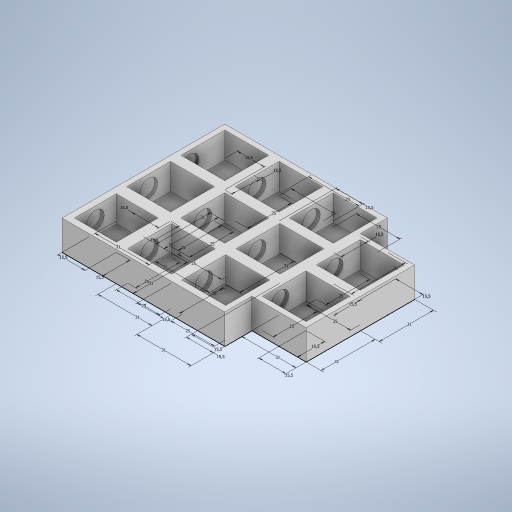
# Autodesk Inventor part: новая коробка
Saved by Autodesk Inventor 2024.2 (Build 282272000, 272)
## iProperties
Created: 2026-01-06
Part Number: новая коробка
Material: Типовые
Document SubType Name: Modeling
Designer: User
Density: 1 g/cm^3
Appearance: По умолчанию
Author: User
Autodesk Inventor part; units mm, degrees
ref_plane "YZ Plane" through (0, 0, 0) normal (1, 0, 0) x (0, 1, 0)
ref_plane "XZ Plane" through (0, 0, 0) normal (0, 1, 0) x (-1, 0, 0)
ref_plane "XY Plane" through (0, 0, 0) normal (0, 0, 1) x (1, 0, 0)
sketch "Эскиз1" plane through (0, 0, 0) normal (0, 1, 0) x (-1, 0, 0)
  line L0 (-12.5, -12.5) -> (12.5, -12.5)
  line L1 (12.5, -12.5) -> (12.5, 12.5)
  line L2 (12.5, 12.5) -> (-12.5, 12.5)
  line L3 (-12.5, 12.5) -> (-12.5, -12.5)
  line L4 (-12.5, -12.5) -> (12.5, 12.5) construction
  line L5 (12.5, -12.5) -> (-12.5, 12.5) construction
  line L6 (-15.5, -15.5) -> (15.5, -15.5)
  line L7 (15.5, -15.5) -> (15.5, 15.5)
  line L8 (15.5, 15.5) -> (-15.5, 15.5)
  line L9 (-15.5, 15.5) -> (-15.5, -15.5)
  line L10 (-15.5, -15.5) -> (15.5, 15.5) construction
  line L11 (15.5, -15.5) -> (-15.5, 15.5) construction
  line L12 (15.5, 15.5) -> (46.5, 15.5)
  line L13 (46.5, 15.5) -> (46.5, -15.5)
  line L14 (46.5, -15.5) -> (15.5, -15.5)
  line L15 (15.5, -15.5) -> (15.5, 15.5)
  line L16 (-15.5, 15.5) -> (-46.5, 15.5)
  line L17 (-46.5, 15.5) -> (-46.5, -15.5)
  line L18 (-46.5, -15.5) -> (-15.5, -15.5)
  line L19 (-15.5, -15.5) -> (-15.5, 15.5)
  line L20 (46.5, -15.5) -> (13.5, -15.5)
  line L21 (13.5, -15.5) -> (13.5, -46.5)
  line L22 (13.5, -46.5) -> (46.5, -46.5)
  line L23 (46.5, -46.5) -> (46.5, -15.5)
  line L24 (-15.5, -15.5) -> (13.5, -15.5)
  line L25 (13.5, -15.5) -> (13.5, -46.5)
  line L26 (13.5, -46.5) -> (-15.5, -46.5)
  line L27 (-15.5, -46.5) -> (-15.5, -15.5)
  line L28 (-15.5, -15.5) -> (-46.5, -15.5)
  line L29 (-46.5, -15.5) -> (-46.5, -46.5)
  line L30 (-46.5, -46.5) -> (-15.5, -46.5)
  line L31 (-15.5, -46.5) -> (-15.5, -15.5)
  line L32 (46.5, 15.5) -> (15.5, 15.5)
  line L33 (15.5, 15.5) -> (15.5, 46.5)
  line L34 (15.5, 46.5) -> (46.5, 46.5)
  line L35 (46.5, 46.5) -> (46.5, 15.5)
  line L36 (15.5, 46.5) -> (-15.5, 46.5)
  line L37 (-15.5, 46.5) -> (-15.5, 15.5)
  line L38 (-15.5, 15.5) -> (15.5, 15.5)
  line L39 (15.5, 15.5) -> (15.5, 46.5)
  line L40 (-15.5, 46.5) -> (-46.5, 46.5)
  line L41 (-46.5, 46.5) -> (-46.5, 15.5)
  line L42 (-46.5, 15.5) -> (-15.5, 15.5)
  line L43 (-15.5, 15.5) -> (-15.5, 46.5)
  line L44 (-46.5, 0) -> (-77.5, 0)
  line L45 (-77.5, 0) -> (-77.5, -31)
  line L46 (-77.5, -31) -> (-46.5, -31)
  line L47 (-46.5, -31) -> (-46.5, 0)
  line L48 (-46.5, 0) -> (-77.5, 0)
  line L49 (-77.5, 0) -> (-77.5, 31)
  line L50 (-77.5, 31) -> (-46.5, 31)
  line L51 (-46.5, 31) -> (-46.5, 0)
  line L52 (-12.5, 17.9528) -> (12.5, 17.9528)
  line L53 (12.5, 17.9528) -> (12.5, 42.9528)
  line L54 (12.5, 42.9528) -> (-12.5, 42.9528)
  line L55 (-12.5, 42.9528) -> (-12.5, 17.9528)
  line L56 (-12.5, 17.9528) -> (12.5, 42.9528) construction
  line L57 (12.5, 17.9528) -> (-12.5, 42.9528) construction
  line L58 (19.0472, 19.0472) -> (42.9528, 19.0472)
  line L59 (42.9528, 19.0472) -> (42.9528, 42.9528)
  line L60 (42.9528, 42.9528) -> (19.0472, 42.9528)
  line L61 (19.0472, 42.9528) -> (19.0472, 19.0472)
  line L62 (19.0472, 19.0472) -> (42.9528, 42.9528) construction
  line L63 (42.9528, 19.0472) -> (19.0472, 42.9528) construction
  line L64 (-43.5, 17.9528) -> (-18.5, 17.9528)
  line L65 (-18.5, 17.9528) -> (-18.5, 42.9528)
  line L66 (-18.5, 42.9528) -> (-43.5, 42.9528)
  line L67 (-43.5, 42.9528) -> (-43.5, 17.9528)
  line L68 (-43.5, 17.9528) -> (-18.5, 42.9528) construction
  line L69 (-18.5, 17.9528) -> (-43.5, 42.9528) construction
  line L70 (-43.5, -13.0472) -> (-18.5, -13.0472)
  line L71 (-18.5, -13.0472) -> (-18.5, 11.9528)
  line L72 (-18.5, 11.9528) -> (-43.5, 11.9528)
  line L73 (-43.5, 11.9528) -> (-43.5, -13.0472)
  line L74 (-43.5, -13.0472) -> (-18.5, 11.9528) construction
  line L75 (-18.5, -13.0472) -> (-43.5, 11.9528) construction
  line L76 (-43.5, -43.5) -> (-18.5, -43.5)
  line L77 (-18.5, -43.5) -> (-18.5, -18.5)
  line L78 (-18.5, -18.5) -> (-43.5, -18.5)
  line L79 (-43.5, -18.5) -> (-43.5, -43.5)
  line L80 (-43.5, -43.5) -> (-18.5, -18.5) construction
  line L81 (-18.5, -43.5) -> (-43.5, -18.5) construction
  line L82 (18.5, -43.5646) -> (43.5, -43.5646)
  line L83 (43.5, -43.5646) -> (43.5, -18.5)
  line L84 (43.5, -18.5) -> (18.5, -18.5)
  line L85 (18.5, -18.5) -> (18.5, -43.5646)
  line L86 (18.5, -43.5646) -> (43.5, -18.5) construction
  line L87 (43.5, -43.5646) -> (18.5, -18.5) construction
  line L88 (-12.5, -43.5) -> (12.5, -43.5)
  line L89 (12.5, -43.5) -> (12.5, -18.5)
  line L90 (12.5, -18.5) -> (-12.5, -18.5)
  line L91 (-12.5, -18.5) -> (-12.5, -43.5)
  line L92 (-12.5, -43.5) -> (12.5, -18.5) construction
  line L93 (12.5, -43.5) -> (-12.5, -18.5) construction
  line L94 (18.5, -12.5) -> (43.5, -12.5)
  line L95 (43.5, -12.5) -> (43.5, 12.5)
  line L96 (43.5, 12.5) -> (18.5, 12.5)
  line L97 (18.5, 12.5) -> (18.5, -12.5)
  line L98 (18.5, -12.5) -> (43.5, 12.5) construction
  line L99 (43.5, -12.5) -> (18.5, 12.5) construction
  line L100 (-74.5, -28) -> (-49.5, -28)
  line L101 (-49.5, -28) -> (-49.5, -3)
  line L102 (-49.5, -3) -> (-74.5, -3)
  line L103 (-74.5, -3) -> (-74.5, -28)
  line L104 (-74.5, -28) -> (-49.5, -3) construction
  line L105 (-49.5, -28) -> (-74.5, -3) construction
  line L106 (-74.5, 28) -> (-49.5, 28)
  line L107 (-49.5, 28) -> (-49.5, 3)
  line L108 (-49.5, 3) -> (-74.5, 3)
  line L109 (-74.5, 3) -> (-74.5, 28)
  line L110 (-74.5, 28) -> (-49.5, 3) construction
  line L111 (-49.5, 28) -> (-74.5, 3) construction
  point P0 (0, 0)
  point P1 (0, 30.4528)
  point P2 (31, 31)
  point P3 (-31, 30.4528)
  point P4 (-31, -0.5472)
  point P5 (-31, -31)
  point P6 (31, -31.0323)
  point P7 (0, -31)
  point P8 (31, 0)
  point P9 (-62, -15.5)
  point P10 (-62, 0)
  point P11 (-77.5, -15.5)
  point P12 (-62, 15.5)
  point P13 (-62, 31)
  point P14 (-46.5, -31)
  point P15 (46.5, 31)
  point P16 (30, -46.5)
  point P17 (-31, -46.5)
  point P18 (31, 15.5)
  dimension "d0" = 25
  dimension "d1" = 25
  dimension "d2" = 31
  dimension "d3" = 31
  dimension "d4" = 31
  dimension "d5" = 31
  dimension "d6" = 31
  dimension "d7" = 31
  dimension "d8" = 31
  dimension "d9" = 29
  dimension "d10" = 31
  dimension "d11" = 31
  dimension "d12" = 31
  dimension "d13" = 31
  dimension "d14" = 31
  dimension "d15" = 25
  dimension "d16" = 25
  dimension "d17" = 15.5
  dimension "d19" = 25
  dimension "d20" = 15.5
  dimension "d41" = 15.5
  dimension "d42" = 15.5
  dimension "d43" = 15.5
  dimension "d44" = 15.5
  dimension "d45" = 15.5
  dimension "d46" = 15.5
  dimension "d47" = 15.5
  dimension "d48" = 25
  dimension "d49" = 25
  dimension "d50" = 25
  dimension "d51" = 25
  dimension "d52" = 25
  dimension "d53" = 25
  dimension "d54" = 25
  dimension "d55" = 25
  dimension "d56" = 15.5
  dimension "d57" = 15.5
  dimension "d58" = 15.5
  dimension "d59" = 15.5
  dimension "d60" = 15.5
  dimension "d61" = 15.5
  constraints: 224 end point, 44 parallel, 32 midpoint, 22 horizontal, 22 perpendicular, 15 point on line
  measures "d0" distance of L0.end L1.end
  measures "d1" distance of L1.end L2.end
  measures "d2" distance of L6.end L7.end
  measures "d3" distance of L7.end L8.end
  measures "d4" distance of L7.end L12.end
  measures "d5" distance of L32.end L33.end
  measures "d6" distance of L49.end L50.end
  measures "d7" distance of L36.end L40.end
  measures "d8" distance of L33.end L36.end
  measures "d9" distance of L21.end L26.end
  measures "d10" distance of L28.end L29.end
  measures "d11" distance of L48.end L49.end
  measures "d12" distance of L44.end L45.end
  measures "d13" distance of L14.end L7.end
  measures "d14" distance of L18.end L8.end
  measures "d15" distance of L100.end L101.end
  measures "d16" distance of L101.end L102.end
  measures "d17" distance of point (-62, 0) point (-62, -15.5)
  measures "d19" distance of L106.end L107.end
  measures "d20" distance of point (-62, 31) point (-62, 15.5)
  measures "d41" distance of point (46.5, 31) point (31, 31)
  measures "d42" distance from line of L34 point (31, 31)
  measures "d43" distance from line of L13 point (31, 0)
  measures "d44" distance of point (30, -46.5) point (31, -31.032)
  measures "d45" distance from line of L37 point (0, 30.453)
  measures "d46" distance from line of L41 point (-31, 30.453)
  measures "d47" distance from line of L17 point (-31, -0.547)
  measures "d48" distance of L64.end L65.end
  measures "d49" distance of L65.end L66.end
  measures "d50" distance of L53.end L54.end
  measures "d51" distance of L52.end L53.end
  measures "d52" distance of L96.end L94.start
  measures "d53" distance of L88.end L89.end
  measures "d54" distance of L88.start L88.end
  measures "d55" distance of L76.start L76.end
  measures "d56" distance from line of L49 point (-62, 15.5)
  measures "d57" distance of point (-77.5, -15.5) point (-62, -15.5)
  measures "d58" distance of point (-31, -46.5) point (-31, -31)
  measures "d59" distance from line of L27 point (0, -31)
  measures "d60" distance from line of L23 point (31, -31.032)
  measures "d61" distance of point (31, 15.5) point (31, 0)
extrude "Выдавливание1" add sketch "Эскиз1" along normal blind 17
extrude "Выдавливание2" add sketch "Эскиз1" along normal blind 2 contours L3 L2 L1 L0 | L55 L54 L53 L52 | L61 L60 L59 L58 | L67 L66 L65 L64 | L73 L72 L71 L70 | L79 L78 L77 L76 | L85 L84 L83 L82 | L91 L90 L89 L88 | L97 L96 L95 L94 | L103 L102 L101 L100 | L106 L107 L108 L109
sketch "Эскиз2" plane through (-42.9528, 17, 42.9528) normal (1, 0, 0) x (0, 0, -1)
  line L0 (0, -15) -> (23.9055, -15) projected
  line L1 (23.9055, -15) -> (23.9055, 0) projected
  line L2 (0, 0) -> (23.9055, 0) projected
  line L3 (0, -15) -> (0, 0) projected
  line L4 (30.4528, -15) -> (55.4528, -15) projected
  line L5 (55.4528, -15) -> (55.4528, 0) projected
  line L6 (30.4528, 0) -> (55.4528, 0) projected
  line L7 (30.4528, -15) -> (30.4528, 0) projected
  line L8 (61.4528, -15) -> (86.5173, -15) projected
  line L9 (86.5173, -15) -> (86.5173, 0) projected
  line L10 (61.4528, 0) -> (86.5173, 0) projected
  line L11 (61.4528, -15) -> (61.4528, 0) projected
  circle A0 centre (11.9528, -7) radius 5
  line L12 (0, -15) -> (23.9055, -15) projected
  circle A1 centre (42.9528, -7) radius 5
  circle A2 centre (66.5, -7) radius 5
  line L13 (30.4528, -15) -> (55.4528, -15) projected
  point P0 (42.9528, -17)
  point P1 (11.9528, -15)
  point P2 (42.9528, -15)
  dimension "d25" = 10
  dimension "d26" = 8
  dimension "d27" = 10
  dimension "d28" = 10
  dimension "d29" = 8
  dimension "d30" = 8
  constraints: 3 centre point, 2 midpoint
  measures "d25" diameter of A0
  measures "d26" distance of point (11.953, -15) A0.centre
  measures "d27" diameter of A1
  measures "d28" diameter of A2
  measures "d29" distance of point (42.953, -15) A1.centre
  measures "d30" distance from line of L8 A2.centre
extrude "Выдавливание3" cut sketch "Эскиз2" against normal blind 2 contours A0 | A1 | A2
sketch "Эскиз3" plane through (49.5, 17, 28) normal (1, 0, 0) x (0, 0, -1)
  line L0 (10.0472, -15) -> (10.0472, 0) projected
  circle A0 centre (10.0472, -7) radius 5
  line L1 (41.0472, -15) -> (41.0472, 0) projected
  circle A1 centre (41.0472, -7) radius 5
  point P0 (28, -17)
  dimension "d35" = 10
  dimension "d36" = 8
  dimension "d37" = 10
  dimension "d38" = 8
  constraints: 2 centre point, 2 point on line
  measures "d35" diameter of A0
  measures "d36" distance of A0.centre L0.start
  measures "d37" diameter of A1
  measures "d38" distance of A1.centre L1.start
extrude "Выдавливание4" cut sketch "Эскиз3" against normal blind 2
sketch "Эскиз4" plane through (12.5, 17, 17.9528) normal (-1, 0, 0) x (0, 0, 1)
  circle A0 centre (12.5, -7) radius 5
  line L0 (0, -15) -> (25, -15) projected
  circle A1 centre (-17.9528, -7) radius 5
  line L1 (-30.4528, -15) -> (-5.4528, -15) projected
  circle A2 centre (-48.9528, -7) radius 5
  line L2 (-61.4528, -15) -> (-36.4528, -15) projected
  point P0 (-17.9528, -17)
  point P1 (12.5, -15)
  point P2 (-17.9528, -15)
  point P3 (-48.9528, -15)
  dimension "d62" = 10
  dimension "d63" = 8
  dimension "d64" = 10
  dimension "d65" = 8
  dimension "d66" = 10
  dimension "d67" = 8
  constraints: 3 centre point, 3 midpoint
  measures "d62" diameter of A0
  measures "d63" distance of A0.centre point (12.5, -15)
  measures "d64" diameter of A1
  measures "d65" distance of A1.centre point (-17.953, -15)
  measures "d66" diameter of A2
  measures "d67" distance of point (-48.953, -15) A2.centre
extrude "Выдавливание5" cut sketch "Эскиз4" along normal blind 27
sketch "Эскиз5" plane through (18.5, 17, 42.9528) normal (1, 0, 0) x (0, 0, -1)
  circle A0 centre (12.5, -7) radius 5 projected
  circle A1 centre (42.9528, -7) radius 5 projected
  circle A2 centre (73.9528, -7) radius 5 projected
  point P0 (42.9528, -17)
extrude "Выдавливание6" cut sketch "Эскиз5" against normal blind 2
